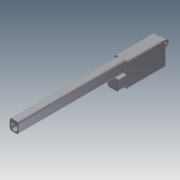
# Autodesk Inventor part: linac body 12in
Saved by Autodesk Inventor 2011 (Build 150239000, 239)
## iProperties
Created: 2011-10-08
Part Number: linac body 12in
Document SubType Name: Modeling
Designer: Matthew
Density: 1 g/cm^3
Author: Matthew
Autodesk Inventor part; units mm, degrees
ref_plane "YZ Plane" through (0, 0, 0) normal (1, 0, 0) x (0, 1, 0)
ref_plane "XZ Plane" through (0, 0, 0) normal (0, 1, 0) x (-1, 0, 0)
ref_plane "XY Plane" through (0, 0, 0) normal (0, 0, 1) x (1, 0, 0)
sketch "Sketch1" plane through (0, 0, 0) normal (0, 0, 1) x (1, 0, 0)
  line L0 (-29.7166, 15.149) -> (9.9074, 15.149)
  line L1 (9.9074, 15.149) -> (9.9074, -58.765)
  line L2 (9.9074, -58.765) -> (-29.7166, -58.765)
  line L3 (-29.7166, -58.765) -> (-29.7166, 15.149)
  point P0 (0, 0)
  dimension "d0" = 39.624
  dimension "d1" = 73.914
  constraints: 8 end point, 2 parallel, 1 horizontal, 1 perpendicular
  measures "d0" distance of L1.end L2.end
  measures "d1" distance of L0.end L1.end
extrude "Extrusion1" add sketch "Sketch1" along normal blind 76.2
sketch "Sketch2" plane through (0, 0, 76.2) normal (0, 0, 1) x (1, 0, 0)
  line L0 (9.9074, 15.149) -> (9.9074, -58.765) projected
  line L1 (-29.7166, 15.149) -> (9.9074, 15.149)
  line L2 (9.9074, 15.149) -> (9.9074, -24.475)
  line L3 (9.9074, -24.475) -> (-29.7166, -24.475)
  line L4 (-29.7166, -24.475) -> (-29.7166, 15.149)
  line L5 (-29.7166, -24.475) -> (-23.3666, -24.475)
  line L6 (-23.3666, -24.475) -> (-23.3666, -18.125)
  line L7 (-23.3666, -18.125) -> (-29.7166, -18.125)
  line L8 (-29.7166, -18.125) -> (-29.7166, -24.475)
  line L9 (-23.3666, -18.125) -> (3.5574, -18.125)
  line L10 (3.5574, -18.125) -> (3.5574, 15.149)
  line L11 (3.5574, 15.149) -> (-23.3666, 15.149)
  line L12 (-23.3666, 15.149) -> (-23.3666, -18.125)
  point P0 (0, 0)
  dimension "d4" = 39.624
  dimension "d5" = 6.35
  dimension "d6" = 6.35
  dimension "d7" = 26.924
  constraints: 24 end point, 6 parallel, 3 horizontal, 3 perpendicular, 2 point on line
  measures "d4" distance of L1.end L2.end
  measures "d5" distance of L7.end L6.end
  measures "d6" distance of L6.end L5.end
  measures "d7" distance of L11.end L10.end
extrude "Extrusion2" add sketch "Sketch2" along normal blind 162.56 contours L10 L9 L12 L1
sketch "Sketch3" plane through (0, 0, 238.76) normal (0, 0, 1) x (1, 0, 0)
  line L0 (-23.3666, 15.149) -> (3.5574, -18.125)
  line L1 (3.5574, 15.149) -> (-23.3666, -18.125)
  circle A0 centre (-9.9046, -1.488) radius 9.906
  point P0 (0, 0)
  dimension "d10" = 19.812
  constraints: 4 end point, 1 centre point, 1 midpoint
  measures "d10" diameter of A0
extrude "Extrusion3" cut sketch "Sketch3" against normal blind 203.2
sketch "Sketch4" plane through (0, 0, 76.2) normal (0, 0, 1) x (1, 0, 0)
  line L0 (3.5574, 15.149) -> (3.5574, -18.125) projected
  line L1 (3.5574, -18.125) -> (-23.3666, -18.125) projected
  line L2 (-23.3666, -18.125) -> (-23.3666, 15.149) projected
  line L3 (-29.7166, 15.149) -> (-23.3666, 15.149) projected
  line L4 (-29.7166, -58.765) -> (-29.7166, 15.149) projected
  line L5 (9.9074, -58.765) -> (-29.7166, -58.765) projected
  line L6 (9.9074, 15.149) -> (9.9074, -58.765) projected
  line L7 (3.5574, 15.149) -> (9.9074, 15.149) projected
  point P0 (0, 0)
extrude "Extrusion4" cut sketch "Sketch4" against normal blind 25.4
sketch "Sketch5" plane through (0, 0, 50.8) normal (0, 0, 1) x (1, 0, 0)
  line L0 (-26.5416, -21.808) -> (6.7324, -21.808)
  line L1 (6.7324, -21.808) -> (6.7324, -55.082)
  line L2 (6.7324, -55.082) -> (-26.5416, -55.082)
  line L3 (-26.5416, -55.082) -> (-26.5416, -21.808)
  point P0 (0, 0)
  dimension "d15" = 33.274
  constraints: 8 end point, 2 parallel, 1 horizontal, 1 perpendicular
  measures "d15" distance of L0.end L1.end
extrude "Extrusion5" add sketch "Sketch5" along normal blind 88.9
sketch "Sketch6" plane through (0, 0, 50.8) normal (0, 0, 1) x (1, 0, 0)
  line L0 (6.7324, -21.808) -> (6.7324, -55.082) projected
  line L1 (6.7324, -55.082) -> (-26.5416, -55.082) projected
  line L2 (-26.5416, -55.082) -> (-26.5416, -21.808) projected
  line L3 (-26.5416, -21.808) -> (6.7324, -21.808) projected
  line L4 (3.5574, -18.125) -> (-23.3666, -18.125) projected
  line L5 (-23.3666, -18.125) -> (-23.3666, 15.149) projected
  line L6 (-29.7166, 15.149) -> (-23.3666, 15.149) projected
  line L7 (-29.7166, -58.765) -> (-29.7166, 15.149) projected
  line L8 (9.9074, -58.765) -> (-29.7166, -58.765) projected
  line L9 (9.9074, 15.149) -> (9.9074, -58.765) projected
  line L10 (3.5574, 15.149) -> (9.9074, 15.149) projected
  line L11 (3.5574, 15.149) -> (3.5574, -18.125) projected
  point P0 (0, 0)
extrude "Extrusion6" add sketch "Sketch6" along normal blind 25.4
sketch "Sketch7" plane through (0, 0, 0) normal (0, 0, -1) x (-1, 0, 0)
  line L0 (-9.9074, 15.149) -> (-9.9074, -58.765) projected
  line L1 (29.7166, -58.765) -> (29.7166, 15.149) projected
  line L2 (-9.9074, 15.149) -> (29.7166, -24.475)
  line L3 (-9.9074, 15.149) -> (46.1294, 15.149) construction
  line L4 (29.7166, 15.149) -> (-9.9074, -24.475)
  line L5 (1.0146, 4.227) -> (18.7946, 4.227)
  line L6 (1.0146, 4.227) -> (18.7946, 4.227)
  line L7 (18.7946, 4.227) -> (18.7946, -13.553)
  line L8 (18.7946, -13.553) -> (1.0146, -13.553)
  line L9 (1.0146, -13.553) -> (1.0146, 4.227)
  point P0 (0, 0)
  dimension "d20" = 45
  dimension "d21" = 17.78
  constraints: 16 end point, 5 point on line, 3 parallel, 2 horizontal, 2 perpendicular, 1 equal length
  measures "d20" angle of L2 L3
  measures "d21" distance of L5.start L5.end
extrude "Extrusion7" add sketch "Sketch7" along normal blind 12.7 contours L5 L4 L2 | L2 L4 L9 | L4 L2 L8 | L4 L7 L2
sketch "Sketch8" plane through (-18.7946, -13.553, 0) normal (-1, 0, 0) x (0, 0, 1)
  line L0 (-12.7, 17.78) -> (-12.7, 0) projected
  circle A0 centre (-12.7, 8.89) radius 3.175
  point P0 (0, 13.553)
  dimension "d24" = 6.35
  constraints: 1 centre point, 1 midpoint
  measures "d24" diameter of A0
extrude "Extrusion8" cut sketch "Sketch8" against normal blind 25.4
sketch "Sketch9" plane through (-1.0146, -13.553, 0) normal (1, 0, 0) x (0, 0, -1)
  arc A0 (12.7, 12.065) -> (12.7, 5.715) centre (12.7, 8.89) ccw projected
  circle A1 centre (12.7, 8.89) radius 3.175
  circle A2 centre (12.7, 8.89) radius 8.89
  point P0 (0, 13.553)
  constraints: 2 coincident, 1 centre point, 1 vertical alignment, 2 other
extrude "Extrusion9" add sketch "Sketch9" against normal blind 17.78
sketch "Sketch10" plane through (0, 0, 76.2) normal (0, 0, 1) x (1, 0, 0)
  line L0 (-26.5416, -55.082) -> (6.7324, -55.082) projected
  line L1 (-26.5416, -21.808) -> (-26.5416, -55.082) projected
  line L2 (6.7324, -21.808) -> (-26.5416, -21.808) projected
  line L3 (6.7324, -55.082) -> (6.7324, -21.808) projected
  line L4 (3.5574, -18.125) -> (3.5574, 15.149) projected
  line L5 (-23.3666, -18.125) -> (3.5574, -18.125) projected
  line L6 (-23.3666, 15.149) -> (-23.3666, -18.125) projected
  line L7 (-29.7166, 15.149) -> (-23.3666, 15.149) projected
  line L8 (-29.7166, -58.765) -> (-29.7166, 15.149) projected
  line L9 (9.9074, -58.765) -> (-29.7166, -58.765) projected
  line L10 (9.9074, 15.149) -> (9.9074, -58.765) projected
  line L11 (3.5574, 15.149) -> (9.9074, 15.149) projected
  point P0 (0, 0)
extrude "Extrusion10" add sketch "Sketch10" along normal blind 38.1
fillet "Fillet1" radius 6.35 11 edges at (9.9074, 15.149, 57.15) (-29.7166, 15.149, 57.15) (9.9074, -58.765, 57.15) (-29.7166, -58.765, 57.15) (-26.5416, -55.082, 127) (6.7324, -55.082, 127) (-9.9046, -58.765, 0) (-23.3666, 15.149, 176.53) (3.5574, 15.149, 176.53) (-23.3666, -18.125, 176.53) (3.5574, -18.125, 176.53)
sketch "Sketch11" plane through (0, 0, 238.76) normal (0, 0, 1) x (1, 0, 0)
  line L0 (-17.0166, 15.149) -> (-2.7926, 15.149) projected
  line L1 (-2.7926, -18.125) -> (-17.0166, -18.125) projected
  line L2 (-9.9046, 15.149) -> (-9.9046, -4.663)
  circle A0 centre (-9.9046, -4.663) radius 9.9046
  point P0 (0, 0)
  dimension "d32" = 19.812
  constraints: 2 end point, 1 centre point, 1 coincident, 1 midpoint, 1 perpendicular
  measures "d32" distance of L2.start L2.end
extrude "Extrusion11" cut sketch "Sketch11" against normal blind 101.6
sketch "Sketch12" plane through (0, 0, 238.76) normal (0, 0, 1) x (1, 0, 0)
  arc A0 (-19.6818, -3.0799) -> (-0.1273, -3.0799) centre (-9.9046, -4.663) ccw projected
  arc A1 (-0.1273, -3.0799) -> (-19.6818, -3.0799) centre (-9.9046, -1.488) ccw projected
  circle A2 centre (-9.9046, -1.488) radius 9.906
  circle A3 centre (-9.9046, -4.663) radius 9.9046
  point P0 (0, 0)
  constraints: 2 centre point, 2 coincident, 2 concentric
extrude "Extrusion12" add sketch "Sketch12" against normal blind 228.6 contours A3 A2 | A1 A3
sketch "Sketch13" plane through (0, 0, 238.76) normal (0, 0, 1) x (1, 0, 0)
  arc A0 (-19.6818, -3.0799) -> (-0.1273, -3.0799) centre (-9.9046, -4.663) ccw projected
  arc A1 (-19.6818, -3.0799) -> (-0.1273, -3.0799) centre (-9.9046, -1.488) ccw projected
  circle A2 centre (-9.9046, -4.663) radius 9.9046
  point P0 (0, 0)
  constraints: 1 centre point, 1 coincident
extrude "Extrusion13" cut sketch "Sketch13" against normal blind 101.6 contours A2 A1
sketch "Sketch14" plane through (0, 0, 238.76) normal (0, 0, 1) x (1, 0, 0)
  circle A0 centre (-9.9046, -4.663) radius 9.9046 projected
  arc A1 (-2.7926, -18.125) -> (3.5574, -11.775) centre (-2.7926, -11.775) ccw projected
  line L0 (3.5574, 8.799) -> (3.5574, -11.775) projected
  arc A2 (3.5574, 8.799) -> (-2.7926, 15.149) centre (-2.7926, 8.799) ccw projected
  line L1 (-17.0166, 15.149) -> (-2.7926, 15.149) projected
  arc A3 (-17.0166, 15.149) -> (-23.3666, 8.799) centre (-17.0166, 8.799) ccw projected
  line L2 (-23.3666, -11.775) -> (-23.3666, 8.799) projected
  arc A4 (-23.3666, -11.775) -> (-17.0166, -18.125) centre (-17.0166, -11.775) ccw projected
  line L3 (-2.7926, -18.125) -> (-17.0166, -18.125) projected
  point P0 (0, 0)
extrude "Extrusion14" add sketch "Sketch14" along normal blind 203.2
body "Solid1"
